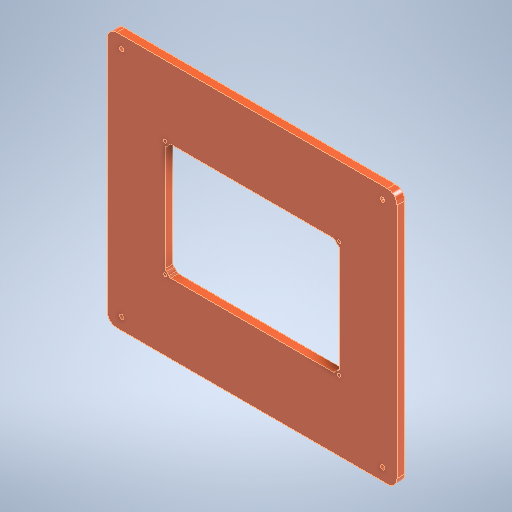
# Autodesk Inventor part: BERÇO GREE
Saved by Autodesk Inventor 2026 (Build 300175050, 175E)
## iProperties
Created: 2025-08-08
Part Number: BERÇO GREE
Material: Genérico
Document SubType Name: Modeling
Designer: Kedson Neves
Density: 1 g/cm^3
Appearance: Suave - Laranja claro
Author: Kedson Neves
Autodesk Inventor part; units mm, degrees
(part 1 of 6)
ref_plane "YZ Plane" through (0, 0, 0) normal (1, 0, 0) x (0, 1, 0)
ref_plane "XZ Plane" through (0, 0, 0) normal (0, 1, 0) x (-1, 0, 0)
ref_plane "XY Plane" through (0, 0, 0) normal (0, 0, 1) x (1, 0, 0)
sketch "Esboço1" plane through (0, 0, 0) normal (0, 0, 1) x (1, 0, 0)
  line L0 (-125.1552, 100.0222) -> (124.8448, 100.0222)
  line L1 (-0.1552, 100.0222) -> (-0.1552, -99.9778)
  line L2 (124.8448, -99.9778) -> (-125.1552, -99.9778)
  line L3 (-150.1552, -132.4778) -> (149.8448, -132.4778)
  line L4 (149.8448, -132.4778) -> (149.8448, 132.5222)
  line L5 (149.8448, 132.5222) -> (-150.1552, 132.5222)
  line L6 (-150.1552, 132.5222) -> (-150.1552, -132.4778)
  line L7 (-150.1552, -132.4778) -> (149.8448, 132.5222) construction
  line L8 (149.8448, -132.4778) -> (-150.1552, 132.5222) construction
  circle A0 centre (-135.1552, 120.0222) radius 1.621
  circle A1 centre (134.8448, 120.0222) radius 1.621
  circle A2 centre (134.8448, -119.9778) radius 1.621
  circle A3 centre (-135.1552, -119.9778) radius 1.621
  point P0 (0, 0)
  point P1 (-0.1552, 0.0222)
  dimension "d0" = 300
  dimension "d1" = 265
  constraints: 18 end point, 4 centre point, 4 midpoint, 2 parallel, 1 horizontal, 1 perpendicular
  measures "d0" distance of L4.end L5.end
  measures "d1" distance of L5.end L3.start
extrude "Extrusão1" add sketch "Esboço1" along normal blind 8
sketch "Esboço2" plane through (0, 0, 8) normal (0, 0, 1) x (1, 0, 0)
  circle A0 centre (-135.1552, 120.0222) radius 1.621 projected
  circle A1 centre (134.8448, 120.0222) radius 1.621 projected
  circle A2 centre (134.8448, -119.9778) radius 1.621 projected
  circle A3 centre (-135.1552, -119.9778) radius 1.621 projected
  point P0 (0, 0)
  constraints: 4 coincident
hole "Furo1" at (-135.1552, 120.0222, 8) at (134.8448, 120.0222, 8) at (134.8448, -119.9778, 8) at (-135.1552, -119.9778, 8) direction (0, 0, -1) diameter 4.5 end through all clearance for "Countersunk Flat Head Screw ISO 2009/7046" size "M4" standard "ISO"
fillet "Arredondamento1" radius 10 4 edges at (-150.1552, -132.4778, 4) (149.8448, -132.4778, 4) (149.8448, 132.5222, 4) (-150.1552, 132.5222, 4)
sketch "Esboço3" plane through (0, 0, 8) normal (0, 0, 1) x (1, 0, 0)
  line L0 (94.8475, -64.9778) -> (94.8475, 65.0222) projected
  line L1 (94.8475, 65.0222) -> (-95.1577, 65.0222) projected
  line L2 (-95.1577, 65.0222) -> (-95.1577, -64.9778) projected
  line L3 (-95.1577, -64.9778) -> (94.8475, -64.9778) projected
  line L4 (91.8485, 60.0222) -> (91.8482, 59.9873) projected
  line L5 (91.8482, 59.9873) -> (91.8473, 59.9524) projected
  line L6 (91.8473, 59.9524) -> (91.8457, 59.9175) projected
  line L7 (91.8457, 59.9175) -> (91.8436, 59.8827) projected
  line L8 (91.8436, 59.8827) -> (91.8409, 59.8479) projected
  line L9 (91.8409, 59.8479) -> (91.8375, 59.8131) projected
  line L10 (91.8375, 59.8131) -> (91.8336, 59.7785) projected
  line L11 (91.8336, 59.7785) -> (91.829, 59.7439) projected
  line L12 (91.829, 59.7439) -> (91.8239, 59.7093) projected
  line L13 (91.8239, 59.7093) -> (91.8181, 59.6749) projected
  line L14 (91.8181, 59.6749) -> (91.8117, 59.6406) projected
  line L15 (91.8117, 59.6406) -> (91.8048, 59.6064) projected
  line L16 (91.8048, 59.6064) -> (91.7972, 59.5723) projected
  line L17 (91.7972, 59.5723) -> (91.7891, 59.5384) projected
  line L18 (91.7891, 59.5384) -> (91.7803, 59.5046) projected
  line L19 (91.7803, 59.5046) -> (91.771, 59.4709) projected
  line L20 (91.771, 59.4709) -> (91.7611, 59.4375) projected
  line L21 (91.7611, 59.4375) -> (91.7506, 59.4042) projected
  line L22 (91.7506, 59.4042) -> (91.7395, 59.3711) projected
  line L23 (91.7395, 59.3711) -> (91.7279, 59.3382) projected
  line L24 (91.7279, 59.3382) -> (91.7156, 59.3055) projected
  line L25 (91.7156, 59.3055) -> (91.7028, 59.273) projected
  line L26 (91.7028, 59.273) -> (91.6895, 59.2407) projected
  line L27 (91.6895, 59.2407) -> (91.6756, 59.2087) projected
  line L28 (91.6756, 59.2087) -> (91.6611, 59.177) projected
  line L29 (91.6611, 59.177) -> (91.6461, 59.1455) projected
  line L30 (91.6461, 59.1455) -> (91.6305, 59.1142) projected
  line L31 (91.6305, 59.1142) -> (91.6144, 59.0833) projected
  line L32 (91.6144, 59.0833) -> (91.5977, 59.0526) projected
  line L33 (91.5977, 59.0526) -> (91.5805, 59.0222) projected
  line L34 (91.5805, 59.0222) -> (91.5628, 58.9921) projected
  line L35 (91.5628, 58.9921) -> (91.5446, 58.9624) projected
  line L36 (91.5446, 58.9624) -> (91.5258, 58.9329) projected
  line L37 (91.5258, 58.9329) -> (91.5066, 58.9038) projected
  line L38 (91.5066, 58.9038) -> (91.4868, 58.8751) projected
  line L39 (91.4868, 58.8751) -> (91.4665, 58.8466) projected
  line L40 (91.4665, 58.8466) -> (91.4458, 58.8186) projected
  line L41 (91.4458, 58.8186) -> (91.4245, 58.7909) projected
  line L42 (91.4245, 58.7909) -> (91.4028, 58.7636) projected
  line L43 (91.4028, 58.7636) -> (91.3806, 58.7366) projected
  line L44 (91.3806, 58.7366) -> (91.3579, 58.7101) projected
  line L45 (91.3579, 58.7101) -> (91.3348, 58.6839) projected
  line L46 (91.3348, 58.6839) -> (91.3112, 58.6582) projected
  line L47 (91.3112, 58.6582) -> (91.2872, 58.6329) projected
  line L48 (91.2872, 58.6329) -> (91.2627, 58.608) projected
  line L49 (91.2627, 58.608) -> (91.2378, 58.5835) projected
  line L50 (91.2378, 58.5835) -> (91.2125, 58.5595) projected
  line L51 (91.2125, 58.5595) -> (91.1867, 58.5359) projected
  line L52 (91.1867, 58.5359) -> (91.1606, 58.5128) projected
  line L53 (91.1606, 58.5128) -> (91.1341, 58.4901) projected
  line L54 (91.1341, 58.4901) -> (91.1071, 58.4679) projected
  line L55 (91.1071, 58.4679) -> (91.0798, 58.4462) projected
  line L56 (91.0798, 58.4462) -> (91.0521, 58.4249) projected
  line L57 (91.0521, 58.4249) -> (91.0241, 58.4042) projected
  line L58 (91.0241, 58.4042) -> (90.9956, 58.3839) projected
  line L59 (90.9956, 58.3839) -> (90.9669, 58.3641) projected
  line L60 (90.9669, 58.3641) -> (90.9378, 58.3449) projected
  line L61 (90.9378, 58.3449) -> (90.9083, 58.3261) projected
  line L62 (90.9083, 58.3261) -> (90.8786, 58.3079) projected
  line L63 (90.8786, 58.3079) -> (90.8485, 58.2902) projected
  line L64 (90.8485, 58.2902) -> (90.8181, 58.273) projected
  line L65 (90.8181, 58.273) -> (90.7874, 58.2563) projected
  line L66 (90.7874, 58.2563) -> (90.7565, 58.2402) projected
  line L67 (90.7565, 58.2402) -> (90.7252, 58.2246) projected
  line L68 (90.7252, 58.2246) -> (90.6937, 58.2096) projected
  line L69 (90.6937, 58.2096) -> (90.662, 58.1951) projected
  line L70 (90.662, 58.1951) -> (90.6299, 58.1812) projected
  line L71 (90.6299, 58.1812) -> (90.5977, 58.1678) projected
  line L72 (90.5977, 58.1678) -> (90.5652, 58.155) projected
  line L73 (90.5652, 58.155) -> (90.5325, 58.1428) projected
  line L74 (90.5325, 58.1428) -> (90.4996, 58.1312) projected
  line L75 (90.4996, 58.1312) -> (90.4665, 58.1201) projected
  line L76 (90.4665, 58.1201) -> (90.4332, 58.1096) projected
  line L77 (90.4332, 58.1096) -> (90.3998, 58.0997) projected
  line L78 (90.3998, 58.0997) -> (90.3661, 58.0904) projected
  line L79 (90.3661, 58.0904) -> (90.3323, 58.0816) projected
  line L80 (90.3323, 58.0816) -> (90.2984, 58.0735) projected
  line L81 (90.2984, 58.0735) -> (90.2643, 58.0659) projected
  line L82 (90.2643, 58.0659) -> (90.2301, 58.059) projected
  line L83 (90.2301, 58.059) -> (90.1958, 58.0526) projected
  line L84 (90.1958, 58.0526) -> (90.1614, 58.0468) projected
  line L85 (90.1614, 58.0468) -> (90.1268, 58.0417) projected
  line L86 (90.1268, 58.0417) -> (90.0922, 58.0371) projected
  line L87 (90.0922, 58.0371) -> (90.0575, 58.0332) projected
  line L88 (90.0575, 58.0332) -> (90.0228, 58.0298) projected
  line L89 (90.0228, 58.0298) -> (89.988, 58.0271) projected
  line L90 (89.988, 58.0271) -> (89.9532, 58.0249) projected
  line L91 (89.9532, 58.0249) -> (89.9183, 58.0234) projected
  line L92 (89.9183, 58.0234) -> (89.8834, 58.0225) projected
  line L93 (89.8834, 58.0225) -> (89.8485, 58.0222) projected
  line L94 (89.8485, 58.0222) -> (89.8136, 58.0225) projected
  line L95 (89.8136, 58.0225) -> (89.7787, 58.0234) projected
  line L96 (89.7787, 58.0234) -> (89.7438, 58.0249) projected
  line L97 (89.7438, 58.0249) -> (89.709, 58.0271) projected
  line L98 (89.709, 58.0271) -> (89.6742, 58.0298) projected
  line L99 (89.6742, 58.0298) -> (89.6394, 58.0332) projected
  line L100 (89.6394, 58.0332) -> (89.6047, 58.0371) projected
  line L101 (89.6047, 58.0371) -> (89.5701, 58.0417) projected
  line L102 (89.5701, 58.0417) -> (89.5356, 58.0468) projected
  line L103 (89.5356, 58.0468) -> (89.5012, 58.0526) projected
  line L104 (89.5012, 58.0526) -> (89.4669, 58.059) projected
  line L105 (89.4669, 58.059) -> (89.4327, 58.0659) projected
  line L106 (89.4327, 58.0659) -> (89.3986, 58.0735) projected
  line L107 (89.3986, 58.0735) -> (89.3646, 58.0816) projected
  line L108 (89.3646, 58.0816) -> (89.3308, 58.0904) projected
  line L109 (89.3308, 58.0904) -> (89.2972, 58.0997) projected
  line L110 (89.2972, 58.0997) -> (89.2637, 58.1096) projected
  line L111 (89.2637, 58.1096) -> (89.2305, 58.1201) projected
  line L112 (89.2305, 58.1201) -> (89.1973, 58.1312) projected
  line L113 (89.1973, 58.1312) -> (89.1644, 58.1428) projected
  line L114 (89.1644, 58.1428) -> (89.1317, 58.155) projected
  line L115 (89.1317, 58.155) -> (89.0993, 58.1678) projected
  line L116 (89.0993, 58.1678) -> (89.067, 58.1812) projected
  line L117 (89.067, 58.1812) -> (89.035, 58.1951) projected
  line L118 (89.035, 58.1951) -> (89.0032, 58.2096) projected
  line L119 (89.0032, 58.2096) -> (88.9717, 58.2246) projected
  line L120 (88.9717, 58.2246) -> (88.9405, 58.2402) projected
  line L121 (88.9405, 58.2402) -> (88.9095, 58.2563) projected
  line L122 (88.9095, 58.2563) -> (88.8789, 58.273) projected
  line L123 (88.8789, 58.273) -> (88.8485, 58.2902) projected
  line L124 (88.8485, 58.2902) -> (88.8184, 58.3079) projected
  line L125 (88.8184, 58.3079) -> (88.7886, 58.3261) projected
  line L126 (88.7886, 58.3261) -> (88.7592, 58.3449) projected
  line L127 (88.7592, 58.3449) -> (88.7301, 58.3641) projected
  line L128 (88.7301, 58.3641) -> (88.7013, 58.3839) projected
  line L129 (88.7013, 58.3839) -> (88.6729, 58.4042) projected
  line L130 (88.6729, 58.4042) -> (88.6449, 58.4249) projected
  line L131 (88.6449, 58.4249) -> (88.6172, 58.4462) projected
  line L132 (88.6172, 58.4462) -> (88.5898, 58.4679) projected
  line L133 (88.5898, 58.4679) -> (88.5629, 58.4901) projected
  line L134 (88.5629, 58.4901) -> (88.5364, 58.5128) projected
  line L135 (88.5364, 58.5128) -> (88.5102, 58.5359) projected
  line L136 (88.5102, 58.5359) -> (88.4845, 58.5595) projected
  line L137 (88.4845, 58.5595) -> (88.4592, 58.5835) projected
  line L138 (88.4592, 58.5835) -> (88.4343, 58.608) projected
  line L139 (88.4343, 58.608) -> (88.4098, 58.6329) projected
  line L140 (88.4098, 58.6329) -> (88.3858, 58.6582) projected
  line L141 (88.3858, 58.6582) -> (88.3622, 58.6839) projected
  line L142 (88.3622, 58.6839) -> (88.3391, 58.7101) projected
  line L143 (88.3391, 58.7101) -> (88.3164, 58.7366) projected
  line L144 (88.3164, 58.7366) -> (88.2942, 58.7636) projected
  line L145 (88.2942, 58.7636) -> (88.2725, 58.7909) projected
  line L146 (88.2725, 58.7909) -> (88.2512, 58.8186) projected
  line L147 (88.2512, 58.8186) -> (88.2305, 58.8466) projected
  line L148 (88.2305, 58.8466) -> (88.2102, 58.8751) projected
  line L149 (88.2102, 58.8751) -> (88.1904, 58.9038) projected
  line L150 (88.1904, 58.9038) -> (88.1711, 58.9329) projected
  line L151 (88.1711, 58.9329) -> (88.1524, 58.9624) projected
  line L152 (88.1524, 58.9624) -> (88.1342, 58.9921) projected
  line L153 (88.1342, 58.9921) -> (88.1164, 59.0222) projected
  line L154 (88.1164, 59.0222) -> (88.0992, 59.0526) projected
  line L155 (88.0992, 59.0526) -> (88.0826, 59.0833) projected
  line L156 (88.0826, 59.0833) -> (88.0665, 59.1142) projected
  line L157 (88.0665, 59.1142) -> (88.0509, 59.1455) projected
  line L158 (88.0509, 59.1455) -> (88.0359, 59.177) projected
  line L159 (88.0359, 59.177) -> (88.0214, 59.2087) projected
  line L160 (88.0214, 59.2087) -> (88.0075, 59.2407) projected
  line L161 (88.0075, 59.2407) -> (87.9941, 59.273) projected
  line L162 (87.9941, 59.273) -> (87.9813, 59.3055) projected
  line L163 (87.9813, 59.3055) -> (87.9691, 59.3382) projected
  line L164 (87.9691, 59.3382) -> (87.9575, 59.3711) projected
  line L165 (87.9575, 59.3711) -> (87.9464, 59.4042) projected
  line L166 (87.9464, 59.4042) -> (87.9359, 59.4375) projected
  line L167 (87.9359, 59.4375) -> (87.926, 59.4709) projected
  line L168 (87.926, 59.4709) -> (87.9166, 59.5046) projected
  line L169 (87.9166, 59.5046) -> (87.9079, 59.5384) projected
  line L170 (87.9079, 59.5384) -> (87.8997, 59.5723) projected
  line L171 (87.8997, 59.5723) -> (87.8922, 59.6064) projected
  line L172 (87.8922, 59.6064) -> (87.8852, 59.6406) projected
  line L173 (87.8852, 59.6406) -> (87.8789, 59.6749) projected
  line L174 (87.8789, 59.6749) -> (87.8731, 59.7093) projected
  line L175 (87.8731, 59.7093) -> (87.868, 59.7439) projected
  line L176 (87.868, 59.7439) -> (87.8634, 59.7785) projected
  line L177 (87.8634, 59.7785) -> (87.8594, 59.8131) projected
  line L178 (87.8594, 59.8131) -> (87.8561, 59.8479) projected
  line L179 (87.8561, 59.8479) -> (87.8534, 59.8827) projected
  line L180 (87.8534, 59.8827) -> (87.8512, 59.9175) projected
  line L181 (87.8512, 59.9175) -> (87.8497, 59.9524) projected
  line L182 (87.8497, 59.9524) -> (87.8488, 59.9873) projected
  line L183 (87.8488, 59.9873) -> (87.8485, 60.0222) projected
  line L184 (87.8485, 60.0222) -> (87.8488, 60.0571) projected
  line L185 (87.8488, 60.0571) -> (87.8497, 60.092) projected
  line L186 (87.8497, 60.092) -> (87.8512, 60.1269) projected
  line L187 (87.8512, 60.1269) -> (87.8534, 60.1617) projected
  line L188 (87.8534, 60.1617) -> (87.8561, 60.1965) projected
  line L189 (87.8561, 60.1965) -> (87.8594, 60.2313) projected
  line L190 (87.8594, 60.2313) -> (87.8634, 60.2659) projected
  line L191 (87.8634, 60.2659) -> (87.868, 60.3005) projected
  line L192 (87.868, 60.3005) -> (87.8731, 60.3351) projected
  line L193 (87.8731, 60.3351) -> (87.8789, 60.3695) projected
  line L194 (87.8789, 60.3695) -> (87.8852, 60.4038) projected
  line L195 (87.8852, 60.4038) -> (87.8922, 60.438) projected
  line L196 (87.8922, 60.438) -> (87.8997, 60.4721) projected
  line L197 (87.8997, 60.4721) -> (87.9079, 60.506) projected
  line L198 (87.9079, 60.506) -> (87.9166, 60.5398) projected
  line L199 (87.9166, 60.5398) -> (87.926, 60.5735) projected
  line L200 (87.926, 60.5735) -> (87.9359, 60.6069) projected
  line L201 (87.9359, 60.6069) -> (87.9464, 60.6402) projected
  line L202 (87.9464, 60.6402) -> (87.9575, 60.6733) projected
  line L203 (87.9575, 60.6733) -> (87.9691, 60.7062) projected
  line L204 (87.9691, 60.7062) -> (87.9813, 60.7389) projected
  line L205 (87.9813, 60.7389) -> (87.9941, 60.7714) projected
  line L206 (87.9941, 60.7714) -> (88.0075, 60.8037) projected
  line L207 (88.0075, 60.8037) -> (88.0214, 60.8357) projected
  line L208 (88.0214, 60.8357) -> (88.0359, 60.8674) projected
  line L209 (88.0359, 60.8674) -> (88.0509, 60.8989) projected
  line L210 (88.0509, 60.8989) -> (88.0665, 60.9302) projected
  line L211 (88.0665, 60.9302) -> (88.0826, 60.9611) projected
  line L212 (88.0826, 60.9611) -> (88.0992, 60.9918) projected
  line L213 (88.0992, 60.9918) -> (88.1164, 61.0222) projected
  line L214 (88.1164, 61.0222) -> (88.1342, 61.0523) projected
  line L215 (88.1342, 61.0523) -> (88.1524, 61.082) projected
  line L216 (88.1524, 61.082) -> (88.1711, 61.1115) projected
  line L217 (88.1711, 61.1115) -> (88.1904, 61.1406) projected
  line L218 (88.1904, 61.1406) -> (88.2102, 61.1694) projected
  line L219 (88.2102, 61.1694) -> (88.2305, 61.1978) projected
  line L220 (88.2305, 61.1978) -> (88.2512, 61.2258) projected
  line L221 (88.2512, 61.2258) -> (88.2725, 61.2535) projected
  line L222 (88.2725, 61.2535) -> (88.2942, 61.2808) projected
  line L223 (88.2942, 61.2808) -> (88.3164, 61.3078) projected
  line L224 (88.3164, 61.3078) -> (88.3391, 61.3343) projected
  line L225 (88.3391, 61.3343) -> (88.3622, 61.3605) projected
  line L226 (88.3622, 61.3605) -> (88.3858, 61.3862) projected
  line L227 (88.3858, 61.3862) -> (88.4098, 61.4115) projected
  line L228 (88.4098, 61.4115) -> (88.4343, 61.4364) projected
  line L229 (88.4343, 61.4364) -> (88.4592, 61.4609) projected
  line L230 (88.4592, 61.4609) -> (88.4845, 61.4849) projected
  line L231 (88.4845, 61.4849) -> (88.5102, 61.5085) projected
  line L232 (88.5102, 61.5085) -> (88.5364, 61.5316) projected
  line L233 (88.5364, 61.5316) -> (88.5629, 61.5543) projected
  line L234 (88.5629, 61.5543) -> (88.5898, 61.5765) projected
  line L235 (88.5898, 61.5765) -> (88.6172, 61.5982) projected
  line L236 (88.6172, 61.5982) -> (88.6449, 61.6195) projected
  line L237 (88.6449, 61.6195) -> (88.6729, 61.6402) projected
  line L238 (88.6729, 61.6402) -> (88.7013, 61.6605) projected
  line L239 (88.7013, 61.6605) -> (88.7301, 61.6803) projected
  line L240 (88.7301, 61.6803) -> (88.7592, 61.6995) projected
  line L241 (88.7592, 61.6995) -> (88.7886, 61.7183) projected
  line L242 (88.7886, 61.7183) -> (88.8184, 61.7365) projected
  line L243 (88.8184, 61.7365) -> (88.8485, 61.7543) projected
  line L244 (88.8485, 61.7543) -> (88.8789, 61.7714) projected
  line L245 (88.8789, 61.7714) -> (88.9095, 61.7881) projected
  line L246 (88.9095, 61.7881) -> (88.9405, 61.8042) projected
  line L247 (88.9405, 61.8042) -> (88.9717, 61.8198) projected
  line L248 (88.9717, 61.8198) -> (89.0032, 61.8348) projected
  line L249 (89.0032, 61.8348) -> (89.035, 61.8493) projected
  line L250 (89.035, 61.8493) -> (89.067, 61.8632) projected
  line L251 (89.067, 61.8632) -> (89.0993, 61.8766) projected
  line L252 (89.0993, 61.8766) -> (89.1317, 61.8894) projected
  line L253 (89.1317, 61.8894) -> (89.1644, 61.9016) projected
  line L254 (89.1644, 61.9016) -> (89.1973, 61.9132) projected
  line L255 (89.1973, 61.9132) -> (89.2305, 61.9243) projected
  line L256 (89.2305, 61.9243) -> (89.2637, 61.9348) projected
  line L257 (89.2637, 61.9348) -> (89.2972, 61.9447) projected
  line L258 (89.2972, 61.9447) -> (89.3308, 61.9541) projected
  line L259 (89.3308, 61.9541) -> (89.3646, 61.9628) projected
  line L260 (89.3646, 61.9628) -> (89.3986, 61.9709) projected
  line L261 (89.3986, 61.9709) -> (89.4327, 61.9785) projected
  line L262 (89.4327, 61.9785) -> (89.4669, 61.9855) projected
  line L263 (89.4669, 61.9855) -> (89.5012, 61.9918) projected
  line L264 (89.5012, 61.9918) -> (89.5356, 61.9976) projected
  line L265 (89.5356, 61.9976) -> (89.5701, 62.0027) projected
  line L266 (89.5701, 62.0027) -> (89.6047, 62.0073) projected
  line L267 (89.6047, 62.0073) -> (89.6394, 62.0112) projected
  line L268 (89.6394, 62.0112) -> (89.6742, 62.0146) projected
  line L269 (89.6742, 62.0146) -> (89.709, 62.0173) projected
  line L270 (89.709, 62.0173) -> (89.7438, 62.0195) projected
  line L271 (89.7438, 62.0195) -> (89.7787, 62.021) projected
  line L272 (89.7787, 62.021) -> (89.8136, 62.0219) projected
  line L273 (89.8136, 62.0219) -> (89.8485, 62.0222) projected
  line L274 (89.8485, 62.0222) -> (89.8834, 62.0219) projected
  line L275 (89.8834, 62.0219) -> (89.9183, 62.021) projected
  line L276 (89.9183, 62.021) -> (89.9532, 62.0195) projected
  line L277 (89.9532, 62.0195) -> (89.988, 62.0173) projected
  line L278 (89.988, 62.0173) -> (90.0228, 62.0146) projected
  line L279 (90.0228, 62.0146) -> (90.0575, 62.0112) projected
  line L280 (90.0575, 62.0112) -> (90.0922, 62.0073) projected
  line L281 (90.0922, 62.0073) -> (90.1268, 62.0027) projected
  line L282 (90.1268, 62.0027) -> (90.1614, 61.9976) projected
  line L283 (90.1614, 61.9976) -> (90.1958, 61.9918) projected
  line L284 (90.1958, 61.9918) -> (90.2301, 61.9855) projected
  line L285 (90.2301, 61.9855) -> (90.2643, 61.9785) projected
  line L286 (90.2643, 61.9785) -> (90.2984, 61.9709) projected
  line L287 (90.2984, 61.9709) -> (90.3323, 61.9628) projected
  line L288 (90.3323, 61.9628) -> (90.3661, 61.9541) projected
  line L289 (90.3661, 61.9541) -> (90.3998, 61.9447) projected
  line L290 (90.3998, 61.9447) -> (90.4332, 61.9348) projected
  line L291 (90.4332, 61.9348) -> (90.4665, 61.9243) projected
  line L292 (90.4665, 61.9243) -> (90.4996, 61.9132) projected
  line L293 (90.4996, 61.9132) -> (90.5325, 61.9016) projected
  line L294 (90.5325, 61.9016) -> (90.5652, 61.8894) projected
  line L295 (90.5652, 61.8894) -> (90.5977, 61.8766) projected
  line L296 (90.5977, 61.8766) -> (90.6299, 61.8632) projected
  line L297 (90.6299, 61.8632) -> (90.662, 61.8493) projected
  line L298 (90.662, 61.8493) -> (90.6937, 61.8348) projected
  line L299 (90.6937, 61.8348) -> (90.7252, 61.8198) projected
  line L300 (90.7252, 61.8198) -> (90.7565, 61.8042) projected
  line L301 (90.7565, 61.8042) -> (90.7874, 61.7881) projected
  line L302 (90.7874, 61.7881) -> (90.8181, 61.7714) projected
  line L303 (90.8181, 61.7714) -> (90.8485, 61.7543) projected
  line L304 (90.8485, 61.7543) -> (90.8786, 61.7365) projected
  line L305 (90.8786, 61.7365) -> (90.9083, 61.7183) projected
  line L306 (90.9083, 61.7183) -> (90.9378, 61.6995) projected
  line L307 (90.9378, 61.6995) -> (90.9669, 61.6803) projected
  line L308 (90.9669, 61.6803) -> (90.9956, 61.6605) projected
  line L309 (90.9956, 61.6605) -> (91.0241, 61.6402) projected
  line L310 (91.0241, 61.6402) -> (91.0521, 61.6195) projected
  line L311 (91.0521, 61.6195) -> (91.0798, 61.5982) projected
  line L312 (91.0798, 61.5982) -> (91.1071, 61.5765) projected
  line L313 (91.1071, 61.5765) -> (91.1341, 61.5543) projected
  line L314 (91.1341, 61.5543) -> (91.1606, 61.5316) projected
  line L315 (91.1606, 61.5316) -> (91.1867, 61.5085) projected
  line L316 (91.1867, 61.5085) -> (91.2125, 61.4849) projected
  line L317 (91.2125, 61.4849) -> (91.2378, 61.4609) projected
  line L318 (91.2378, 61.4609) -> (91.2627, 61.4364) projected
  line L319 (91.2627, 61.4364) -> (91.2872, 61.4115) projected
  line L320 (91.2872, 61.4115) -> (91.3112, 61.3862) projected
  line L321 (91.3112, 61.3862) -> (91.3348, 61.3605) projected
  line L322 (91.3348, 61.3605) -> (91.3579, 61.3343) projected
  line L323 (91.3579, 61.3343) -> (91.3806, 61.3078) projected
  line L324 (91.3806, 61.3078) -> (91.4028, 61.2808) projected
  line L325 (91.4028, 61.2808) -> (91.4245, 61.2535) projected
  line L326 (91.4245, 61.2535) -> (91.4458, 61.2258) projected
  line L327 (91.4458, 61.2258) -> (91.4665, 61.1978) projected
  line L328 (91.4665, 61.1978) -> (91.4868, 61.1694) projected
  line L329 (91.4868, 61.1694) -> (91.5066, 61.1406) projected
  line L330 (91.5066, 61.1406) -> (91.5258, 61.1115) projected
  line L331 (91.5258, 61.1115) -> (91.5446, 61.082) projected
  line L332 (91.5446, 61.082) -> (91.5628, 61.0523) projected
  line L333 (91.5628, 61.0523) -> (91.5805, 61.0222) projected
  line L334 (91.5805, 61.0222) -> (91.5977, 60.9918) projected
  line L335 (91.5977, 60.9918) -> (91.6144, 60.9611) projected
  line L336 (91.6144, 60.9611) -> (91.6305, 60.9302) projected
  line L337 (91.6305, 60.9302) -> (91.6461, 60.8989) projected
  line L338 (91.6461, 60.8989) -> (91.6611, 60.8674) projected
  line L339 (91.6611, 60.8674) -> (91.6756, 60.8357) projected
  line L340 (91.6756, 60.8357) -> (91.6895, 60.8037) projected
  line L341 (91.6895, 60.8037) -> (91.7028, 60.7714) projected
  line L342 (91.7028, 60.7714) -> (91.7156, 60.7389) projected
  line L343 (91.7156, 60.7389) -> (91.7279, 60.7062) projected
  line L344 (91.7279, 60.7062) -> (91.7395, 60.6733) projected
  line L345 (91.7395, 60.6733) -> (91.7506, 60.6402) projected
  line L346 (91.7506, 60.6402) -> (91.7611, 60.6069) projected
  line L347 (91.7611, 60.6069) -> (91.771, 60.5735) projected
  line L348 (91.771, 60.5735) -> (91.7803, 60.5398) projected
  line L349 (91.7803, 60.5398) -> (91.7891, 60.506) projected
  line L350 (91.7891, 60.506) -> (91.7972, 60.4721) projected
  line L351 (91.7972, 60.4721) -> (91.8048, 60.438) projected
  line L352 (91.8048, 60.438) -> (91.8117, 60.4038) projected
  line L353 (91.8117, 60.4038) -> (91.8181, 60.3695) projected
  line L354 (91.8181, 60.3695) -> (91.8239, 60.3351) projected
  line L355 (91.8239, 60.3351) -> (91.829, 60.3005) projected
  line L356 (91.829, 60.3005) -> (91.8336, 60.2659) projected
  line L357 (91.8336, 60.2659) -> (91.8375, 60.2313) projected
  line L358 (91.8375, 60.2313) -> (91.8409, 60.1965) projected
  line L359 (91.8409, 60.1965) -> (91.8436, 60.1617) projected
  line L360 (91.8436, 60.1617) -> (91.8457, 60.1269) projected
  line L361 (91.8457, 60.1269) -> (91.8473, 60.092) projected
  line L362 (91.8473, 60.092) -> (91.8482, 60.0571) projected
  line L363 (91.8482, 60.0571) -> (91.8485, 60.0222) projected
  line L364 (91.8485, -59.9778) -> (91.8482, -60.0127) projected
  line L365 (91.8482, -60.0127) -> (91.8473, -60.0476) projected
  line L366 (91.8473, -60.0476) -> (91.8457, -60.0825) projected
  line L367 (91.8457, -60.0825) -> (91.8436, -60.1173) projected
  line L368 (91.8436, -60.1173) -> (91.8409, -60.1521) projected
  line L369 (91.8409, -60.1521) -> (91.8375, -60.1869) projected
  line L370 (91.8375, -60.1869) -> (91.8336, -60.2215) projected
  line L371 (91.8336, -60.2215) -> (91.829, -60.2562) projected
  line L372 (91.829, -60.2562) -> (91.8239, -60.2907) projected
  line L373 (91.8239, -60.2907) -> (91.8181, -60.3251) projected
  line L374 (91.8181, -60.3251) -> (91.8117, -60.3594) projected
  line L375 (91.8117, -60.3594) -> (91.8048, -60.3936) projected
  line L376 (91.8048, -60.3936) -> (91.7972, -60.4277) projected
  line L377 (91.7972, -60.4277) -> (91.7891, -60.4617) projected
  line L378 (91.7891, -60.4617) -> (91.7803, -60.4954) projected
  line L379 (91.7803, -60.4954) -> (91.771, -60.5291) projected
  line L380 (91.771, -60.5291) -> (91.7611, -60.5626) projected
  line L381 (91.7611, -60.5626) -> (91.7506, -60.5958) projected
  line L382 (91.7506, -60.5958) -> (91.7395, -60.6289) projected
  line L383 (91.7395, -60.6289) -> (91.7279, -60.6618) projected
  line L384 (91.7279, -60.6618) -> (91.7156, -60.6945) projected
  line L385 (91.7156, -60.6945) -> (91.7028, -60.727) projected
  line L386 (91.7028, -60.727) -> (91.6895, -60.7593) projected
  line L387 (91.6895, -60.7593) -> (91.6756, -60.7913) projected
  line L388 (91.6756, -60.7913) -> (91.6611, -60.823) projected
  line L389 (91.6611, -60.823) -> (91.6461, -60.8546) projected
  line L390 (91.6461, -60.8546) -> (91.6305, -60.8858) projected
  line L391 (91.6305, -60.8858) -> (91.6144, -60.9168) projected
  line L392 (91.6144, -60.9168) -> (91.5977, -60.9474) projected
  line L393 (91.5977, -60.9474) -> (91.5805, -60.9778) projected
  line L394 (91.5805, -60.9778) -> (91.5628, -61.0079) projected
  line L395 (91.5628, -61.0079) -> (91.5446, -61.0376) projected
  line L396 (91.5446, -61.0376) -> (91.5258, -61.0671) projected
  line L397 (91.5258, -61.0671) -> (91.5066, -61.0962) projected
  line L398 (91.5066, -61.0962) -> (91.4868, -61.125) projected
  line L399 (91.4868, -61.125) -> (91.4665, -61.1534) projected
  line L400 (91.4665, -61.1534) -> (91.4458, -61.1814) projected
  line L401 (91.4458, -61.1814) -> (91.4245, -61.2091) projected
  line L402 (91.4245, -61.2091) -> (91.4028, -61.2364) projected
  line L403 (91.4028, -61.2364) -> (91.3806, -61.2634) projected
  line L404 (91.3806, -61.2634) -> (91.3579, -61.2899) projected
  line L405 (91.3579, -61.2899) -> (91.3348, -61.3161) projected
  line L406 (91.3348, -61.3161) -> (91.3112, -61.3418) projected
  line L407 (91.3112, -61.3418) -> (91.2872, -61.3671) projected
  line L408 (91.2872, -61.3671) -> (91.2627, -61.392) projected
  line L409 (91.2627, -61.392) -> (91.2378, -61.4165) projected
  line L410 (91.2378, -61.4165) -> (91.2125, -61.4405) projected
  line L411 (91.2125, -61.4405) -> (91.1867, -61.4641) projected
  line L412 (91.1867, -61.4641) -> (91.1606, -61.4872) projected
  line L413 (91.1606, -61.4872) -> (91.1341, -61.5099) projected
  line L414 (91.1341, -61.5099) -> (91.1071, -61.5321) projected
  line L415 (91.1071, -61.5321) -> (91.0798, -61.5538) projected
  line L416 (91.0798, -61.5538) -> (91.0521, -61.5751) projected
  line L417 (91.0521, -61.5751) -> (91.0241, -61.5958) projected
  line L418 (91.0241, -61.5958) -> (90.9956, -61.6161) projected
  line L419 (90.9956, -61.6161) -> (90.9669, -61.6359) projected
  line L420 (90.9669, -61.6359) -> (90.9378, -61.6551) projected
  line L421 (90.9378, -61.6551) -> (90.9083, -61.6739) projected
  line L422 (90.9083, -61.6739) -> (90.8786, -61.6921) projected
  line L423 (90.8786, -61.6921) -> (90.8485, -61.7099) projected
  line L424 (90.8485, -61.7099) -> (90.8181, -61.727) projected
  line L425 (90.8181, -61.727) -> (90.7874, -61.7437) projected
  line L426 (90.7874, -61.7437) -> (90.7565, -61.7598) projected
  line L427 (90.7565, -61.7598) -> (90.7252, -61.7754) projected
  line L428 (90.7252, -61.7754) -> (90.6937, -61.7904) projected
  line L429 (90.6937, -61.7904) -> (90.662, -61.8049) projected
  line L430 (90.662, -61.8049) -> (90.6299, -61.8188) projected
  line L431 (90.6299, -61.8188) -> (90.5977, -61.8322) projected
  line L432 (90.5977, -61.8322) -> (90.5652, -61.845) projected
  line L433 (90.5652, -61.845) -> (90.5325, -61.8572) projected
  line L434 (90.5325, -61.8572) -> (90.4996, -61.8688) projected
  line L435 (90.4996, -61.8688) -> (90.4665, -61.8799) projected
  line L436 (90.4665, -61.8799) -> (90.4332, -61.8904) projected
  line L437 (90.4332, -61.8904) -> (90.3998, -61.9003) projected
  line L438 (90.3998, -61.9003) -> (90.3661, -61.9097) projected
  line L439 (90.3661, -61.9097) -> (90.3323, -61.9184) projected
  line L440 (90.3323, -61.9184) -> (90.2984, -61.9265) projected
  line L441 (90.2984, -61.9265) -> (90.2643, -61.9341) projected
  line L442 (90.2643, -61.9341) -> (90.2301, -61.9411) projected
  line L443 (90.2301, -61.9411) -> (90.1958, -61.9474) projected
  line L444 (90.1958, -61.9474) -> (90.1614, -61.9532) projected
  line L445 (90.1614, -61.9532) -> (90.1268, -61.9583) projected
  line L446 (90.1268, -61.9583) -> (90.0922, -61.9629) projected
  line L447 (90.0922, -61.9629) -> (90.0575, -61.9668) projected
  line L448 (90.0575, -61.9668) -> (90.0228, -61.9702) projected
  line L449 (90.0228, -61.9702) -> (89.988, -61.9729) projected
  line L450 (89.988, -61.9729) -> (89.9532, -61.9751) projected
  line L451 (89.9532, -61.9751) -> (89.9183, -61.9766) projected
  line L452 (89.9183, -61.9766) -> (89.8834, -61.9775) projected
  line L453 (89.8834, -61.9775) -> (89.8485, -61.9778) projected
  line L454 (89.8485, -61.9778) -> (89.8136, -61.9775) projected
  line L455 (89.8136, -61.9775) -> (89.7787, -61.9766) projected
  line L456 (89.7787, -61.9766) -> (89.7438, -61.9751) projected
  line L457 (89.7438, -61.9751) -> (89.709, -61.9729) projected
  line L458 (89.709, -61.9729) -> (89.6742, -61.9702) projected
  line L459 (89.6742, -61.9702) -> (89.6394, -61.9668) projected
  line L460 (89.6394, -61.9668) -> (89.6047, -61.9629) projected
  line L461 (89.6047, -61.9629) -> (89.5701, -61.9583) projected
  line L462 (89.5701, -61.9583) -> (89.5356, -61.9532) projected
  line L463 (89.5356, -61.9532) -> (89.5012, -61.9474) projected
  line L464 (89.5012, -61.9474) -> (89.4669, -61.9411) projected
  line L465 (89.4669, -61.9411) -> (89.4327, -61.9341) projected
  line L466 (89.4327, -61.9341) -> (89.3986, -61.9265) projected
  line L467 (89.3986, -61.9265) -> (89.3646, -61.9184) projected
  line L468 (89.3646, -61.9184) -> (89.3308, -61.9097) projected
  line L469 (89.3308, -61.9097) -> (89.2972, -61.9003) projected
  line L470 (89.2972, -61.9003) -> (89.2637, -61.8904) projected
  line L471 (89.2637, -61.8904) -> (89.2305, -61.8799) projected
  line L472 (89.2305, -61.8799) -> (89.1973, -61.8688) projected
  line L473 (89.1973, -61.8688) -> (89.1644, -61.8572) projected
  line L474 (89.1644, -61.8572) -> (89.1317, -61.845) projected
  line L475 (89.1317, -61.845) -> (89.0993, -61.8322) projected
  line L476 (89.0993, -61.8322) -> (89.067, -61.8188) projected
  line L477 (89.067, -61.8188) -> (89.035, -61.8049) projected
  line L478 (89.035, -61.8049) -> (89.0032, -61.7904) projected
  line L479 (89.0032, -61.7904) -> (88.9717, -61.7754) projected
  line L480 (88.9717, -61.7754) -> (88.9405, -61.7598) projected
  line L481 (88.9405, -61.7598) -> (88.9095, -61.7437) projected
  line L482 (88.9095, -61.7437) -> (88.8789, -61.727) projected
  line L483 (88.8789, -61.727) -> (88.8485, -61.7099) projected
  line L484 (88.8485, -61.7099) -> (88.8184, -61.6921) projected
  line L485 (88.8184, -61.6921) -> (88.7886, -61.6739) projected
  line L486 (88.7886, -61.6739) -> (88.7592, -61.6551) projected
  line L487 (88.7592, -61.6551) -> (88.7301, -61.6359) projected
  line L488 (88.7301, -61.6359) -> (88.7013, -61.6161) projected
  line L489 (88.7013, -61.6161) -> (88.6729, -61.5958) projected
  line L490 (88.6729, -61.5958) -> (88.6449, -61.5751) projected
  line L491 (88.6449, -61.5751) -> (88.6172, -61.5538) projected
  line L492 (88.6172, -61.5538) -> (88.5898, -61.5321) projected
  line L493 (88.5898, -61.5321) -> (88.5629, -61.5099) projected
  line L494 (88.5629, -61.5099) -> (88.5364, -61.4872) projected
  line L495 (88.5364, -61.4872) -> (88.5102, -61.4641) projected
  line L496 (88.5102, -61.4641) -> (88.4845, -61.4405) projected
  line L497 (88.4845, -61.4405) -> (88.4592, -61.4165) projected
  line L498 (88.4592, -61.4165) -> (88.4343, -61.392) projected
  line L499 (88.4343, -61.392) -> (88.4098, -61.3671) projected
  line L500 (88.4098, -61.3671) -> (88.3858, -61.3418) projected
  line L501 (88.3858, -61.3418) -> (88.3622, -61.3161) projected
  line L502 (88.3622, -61.3161) -> (88.3391, -61.2899) projected
  line L503 (88.3391, -61.2899) -> (88.3164, -61.2634) projected
  line L504 (88.3164, -61.2634) -> (88.2942, -61.2364) projected
  line L505 (88.2942, -61.2364) -> (88.2725, -61.2091) projected
  line L506 (88.2725, -61.2091) -> (88.2512, -61.1814) projected
  line L507 (88.2512, -61.1814) -> (88.2305, -61.1534) projected
  line L508 (88.2305, -61.1534) -> (88.2102, -61.125) projected
  line L509 (88.2102, -61.125) -> (88.1904, -61.0962) projected
  line L510 (88.1904, -61.0962) -> (88.1711, -61.0671) projected
  line L511 (88.1711, -61.0671) -> (88.1524, -61.0376) projected
  line L512 (88.1524, -61.0376) -> (88.1342, -61.0079) projected
  line L513 (88.1342, -61.0079) -> (88.1164, -60.9778) projected
  line L514 (88.1164, -60.9778) -> (88.0992, -60.9474) projected
  line L515 (88.0992, -60.9474) -> (88.0826, -60.9168) projected
  line L516 (88.0826, -60.9168) -> (88.0665, -60.8858) projected
  line L517 (88.0665, -60.8858) -> (88.0509, -60.8546) projected
  line L518 (88.0509, -60.8546) -> (88.0359, -60.823) projected
  line L519 (88.0359, -60.823) -> (88.0214, -60.7913) projected
  line L520 (88.0214, -60.7913) -> (88.0075, -60.7593) projected
  line L521 (88.0075, -60.7593) -> (87.9941, -60.727) projected
  line L522 (87.9941, -60.727) -> (87.9813, -60.6945) projected
  line L523 (87.9813, -60.6945) -> (87.9691, -60.6618) projected
  line L524 (87.9691, -60.6618) -> (87.9575, -60.6289) projected
  line L525 (87.9575, -60.6289) -> (87.9464, -60.5958) projected
  line L526 (87.9464, -60.5958) -> (87.9359, -60.5626) projected
  line L527 (87.9359, -60.5626) -> (87.926, -60.5291) projected
  line L528 (87.926, -60.5291) -> (87.9166, -60.4954) projected
  line L529 (87.9166, -60.4954) -> (87.9079, -60.4617) projected
  line L530 (87.9079, -60.4617) -> (87.8997, -60.4277) projected
  line L531 (87.8997, -60.4277) -> (87.8922, -60.3936) projected
  line L532 (87.8922, -60.3936) -> (87.8852, -60.3594) projected
  line L533 (87.8852, -60.3594) -> (87.8789, -60.3251) projected
  line L534 (87.8789, -60.3251) -> (87.8731, -60.2907) projected
  line L535 (87.8731, -60.2907) -> (87.868, -60.2562) projected
  line L536 (87.868, -60.2562) -> (87.8634, -60.2215) projected
  line L537 (87.8634, -60.2215) -> (87.8594, -60.1869) projected
  line L538 (87.8594, -60.1869) -> (87.8561, -60.1521) projected
  line L539 (87.8561, -60.1521) -> (87.8534, -60.1173) projected
  line L540 (87.8534, -60.1173) -> (87.8512, -60.0825) projected
  line L541 (87.8512, -60.0825) -> (87.8497, -60.0476) projected
  line L542 (87.8497, -60.0476) -> (87.8488, -60.0127) projected
  line L543 (87.8488, -60.0127) -> (87.8485, -59.9778) projected
  line L544 (87.8485, -59.9778) -> (87.8488, -59.9429) projected
  line L545 (87.8488, -59.9429) -> (87.8497, -59.908) projected
  line L546 (87.8497, -59.908) -> (87.8512, -59.8731) projected
  line L547 (87.8512, -59.8731) -> (87.8534, -59.8383) projected
  line L548 (87.8534, -59.8383) -> (87.8561, -59.8035) projected
  line L549 (87.8561, -59.8035) -> (87.8594, -59.7688) projected
  line L550 (87.8594, -59.7688) -> (87.8634, -59.7341) projected
  line L551 (87.8634, -59.7341) -> (87.868, -59.6995) projected
  line L552 (87.868, -59.6995) -> (87.8731, -59.6649) projected
  line L553 (87.8731, -59.6649) -> (87.8789, -59.6305) projected
  line L554 (87.8789, -59.6305) -> (87.8852, -59.5962) projected
  line L555 (87.8852, -59.5962) -> (87.8922, -59.562) projected
  line L556 (87.8922, -59.562) -> (87.8997, -59.5279) projected
  line L557 (87.8997, -59.5279) -> (87.9079, -59.494) projected
  line L558 (87.9079, -59.494) -> (87.9166, -59.4602) projected
  line L559 (87.9166, -59.4602) -> (87.926, -59.4265) projected
  line L560 (87.926, -59.4265) -> (87.9359, -59.3931) projected
  line L561 (87.9359, -59.3931) -> (87.9464, -59.3598) projected
  line L562 (87.9464, -59.3598) -> (87.9575, -59.3267) projected
  line L563 (87.9575, -59.3267) -> (87.9691, -59.2938) projected
  line L564 (87.9691, -59.2938) -> (87.9813, -59.2611) projected
  line L565 (87.9813, -59.2611) -> (87.9941, -59.2286) projected
  line L566 (87.9941, -59.2286) -> (88.0075, -59.1963) projected
  line L567 (88.0075, -59.1963) -> (88.0214, -59.1643) projected
  line L568 (88.0214, -59.1643) -> (88.0359, -59.1326) projected
  line L569 (88.0359, -59.1326) -> (88.0509, -59.1011) projected
  line L570 (88.0509, -59.1011) -> (88.0665, -59.0698) projected
  line L571 (88.0665, -59.0698) -> (88.0826, -59.0389) projected
  line L572 (88.0826, -59.0389) -> (88.0992, -59.0082) projected
  line L573 (88.0992, -59.0082) -> (88.1164, -58.9778) projected
  line L574 (88.1164, -58.9778) -> (88.1342, -58.9477) projected
  line L575 (88.1342, -58.9477) -> (88.1524, -58.918) projected
  line L576 (88.1524, -58.918) -> (88.1711, -58.8885) projected
  line L577 (88.1711, -58.8885) -> (88.1904, -58.8594) projected
  line L578 (88.1904, -58.8594) -> (88.2102, -58.8307) projected
  line L579 (88.2102, -58.8307) -> (88.2305, -58.8022) projected
  line L580 (88.2305, -58.8022) -> (88.2512, -58.7742) projected
  line L581 (88.2512, -58.7742) -> (88.2725, -58.7465) projected
  line L582 (88.2725, -58.7465) -> (88.2942, -58.7192) projected
  line L583 (88.2942, -58.7192) -> (88.3164, -58.6922) projected
  line L584 (88.3164, -58.6922) -> (88.3391, -58.6657) projected
  line L585 (88.3391, -58.6657) -> (88.3622, -58.6396) projected
  line L586 (88.3622, -58.6396) -> (88.3858, -58.6138) projected
  line L587 (88.3858, -58.6138) -> (88.4098, -58.5885) projected
  line L588 (88.4098, -58.5885) -> (88.4343, -58.5636) projected
  line L589 (88.4343, -58.5636) -> (88.4592, -58.5391) projected
  line L590 (88.4592, -58.5391) -> (88.4845, -58.5151) projected
  line L591 (88.4845, -58.5151) -> (88.5102, -58.4915) projected
  line L592 (88.5102, -58.4915) -> (88.5364, -58.4684) projected
  line L593 (88.5364, -58.4684) -> (88.5629, -58.4457) projected
  line L594 (88.5629, -58.4457) -> (88.5898, -58.4235) projected
  line L595 (88.5898, -58.4235) -> (88.6172, -58.4018) projected
  line L596 (88.6172, -58.4018) -> (88.6449, -58.3805) projected
  line L597 (88.6449, -58.3805) -> (88.6729, -58.3598) projected
  line L598 (88.6729, -58.3598) -> (88.7013, -58.3395) projected
  line L599 (88.7013, -58.3395) -> (88.7301, -58.3197) projected
  line L600 (88.7301, -58.3197) -> (88.7592, -58.3005) projected
  line L601 (88.7592, -58.3005) -> (88.7886, -58.2817) projected
  line L602 (88.7886, -58.2817) -> (88.8184, -58.2635) projected
  line L603 (88.8184, -58.2635) -> (88.8485, -58.2458) projected
  line L604 (88.8485, -58.2458) -> (88.8789, -58.2286) projected
  line L605 (88.8789, -58.2286) -> (88.9095, -58.2119) projected
  line L606 (88.9095, -58.2119) -> (88.9405, -58.1958) projected
  line L607 (88.9405, -58.1958) -> (88.9717, -58.1802) projected
  line L608 (88.9717, -58.1802) -> (89.0032, -58.1652) projected
  line L609 (89.0032, -58.1652) -> (89.035, -58.1507) projected
  line L610 (89.035, -58.1507) -> (89.067, -58.1368) projected
  line L611 (89.067, -58.1368) -> (89.0993, -58.1234) projected
  line L612 (89.0993, -58.1234) -> (89.1317, -58.1107) projected
  line L613 (89.1317, -58.1107) -> (89.1644, -58.0984) projected
  line L614 (89.1644, -58.0984) -> (89.1973, -58.0868) projected
  line L615 (89.1973, -58.0868) -> (89.2305, -58.0757) projected
  line L616 (89.2305, -58.0757) -> (89.2637, -58.0652) projected
  line L617 (89.2637, -58.0652) -> (89.2972, -58.0553) projected
  line L618 (89.2972, -58.0553) -> (89.3308, -58.046) projected
  line L619 (89.3308, -58.046) -> (89.3646, -58.0372) projected
  line L620 (89.3646, -58.0372) -> (89.3986, -58.0291) projected
  line L621 (89.3986, -58.0291) -> (89.4327, -58.0215) projected
  line L622 (89.4327, -58.0215) -> (89.4669, -58.0146) projected
  line L623 (89.4669, -58.0146) -> (89.5012, -58.0082) projected
  line L624 (89.5012, -58.0082) -> (89.5356, -58.0024) projected
  line L625 (89.5356, -58.0024) -> (89.5701, -57.9973) projected
  line L626 (89.5701, -57.9973) -> (89.6047, -57.9927) projected
  line L627 (89.6047, -57.9927) -> (89.6394, -57.9888) projected
  line L628 (89.6394, -57.9888) -> (89.6742, -57.9854) projected
  line L629 (89.6742, -57.9854) -> (89.709, -57.9827) projected
  line L630 (89.709, -57.9827) -> (89.7438, -57.9806) projected
  line L631 (89.7438, -57.9806) -> (89.7787, -57.979) projected
  line L632 (89.7787, -57.979) -> (89.8136, -57.9781) projected
  line L633 (89.8136, -57.9781) -> (89.8485, -57.9778) projected
  line L634 (89.8485, -57.9778) -> (89.8834, -57.9781) projected
  line L635 (89.8834, -57.9781) -> (89.9183, -57.979) projected
  line L636 (89.9183, -57.979) -> (89.9532, -57.9806) projected
  line L637 (89.9532, -57.9806) -> (89.988, -57.9827) projected
  line L638 (89.988, -57.9827) -> (90.0228, -57.9854) projected
  line L639 (90.0228, -57.9854) -> (90.0575, -57.9888) projected
  line L640 (90.0575, -57.9888) -> (90.0922, -57.9927) projected
  line L641 (90.0922, -57.9927) -> (90.1268, -57.9973) projected
  line L642 (90.1268, -57.9973) -> (90.1614, -58.0024) projected
  line L643 (90.1614, -58.0024) -> (90.1958, -58.0082) projected
  line L644 (90.1958, -58.0082) -> (90.2301, -58.0146) projected
  line L645 (90.2301, -58.0146) -> (90.2643, -58.0215) projected
  line L646 (90.2643, -58.0215) -> (90.2984, -58.0291) projected
  line L647 (90.2984, -58.0291) -> (90.3323, -58.0372) projected
  line L648 (90.3323, -58.0372) -> (90.3661, -58.046) projected
  line L649 (90.3661, -58.046) -> (90.3998, -58.0553) projected
  line L650 (90.3998, -58.0553) -> (90.4332, -58.0652) projected
  line L651 (90.4332, -58.0652) -> (90.4665, -58.0757) projected
  line L652 (90.4665, -58.0757) -> (90.4996, -58.0868) projected
  line L653 (90.4996, -58.0868) -> (90.5325, -58.0984) projected
  line L654 (90.5325, -58.0984) -> (90.5652, -58.1107) projected
  line L655 (90.5652, -58.1107) -> (90.5977, -58.1234) projected
  line L656 (90.5977, -58.1234) -> (90.6299, -58.1368) projected
  line L657 (90.6299, -58.1368) -> (90.662, -58.1507) projected
  line L658 (90.662, -58.1507) -> (90.6937, -58.1652) projected
  line L659 (90.6937, -58.1652) -> (90.7252, -58.1802) projected
  line L660 (90.7252, -58.1802) -> (90.7565, -58.1958) projected
  line L661 (90.7565, -58.1958) -> (90.7874, -58.2119) projected
  line L662 (90.7874, -58.2119) -> (90.8181, -58.2286) projected
  line L663 (90.8181, -58.2286) -> (90.8485, -58.2458) projected
  line L664 (90.8485, -58.2458) -> (90.8786, -58.2635) projected
  line L665 (90.8786, -58.2635) -> (90.9083, -58.2817) projected
  line L666 (90.9083, -58.2817) -> (90.9378, -58.3005) projected
  line L667 (90.9378, -58.3005) -> (90.9669, -58.3197) projected
  line L668 (90.9669, -58.3197) -> (90.9956, -58.3395) projected
  line L669 (90.9956, -58.3395) -> (91.0241, -58.3598) projected
  line L670 (91.0241, -58.3598) -> (91.0521, -58.3805) projected
  line L671 (91.0521, -58.3805) -> (91.0798, -58.4018) projected
  line L672 (91.0798, -58.4018) -> (91.1071, -58.4235) projected
  line L673 (91.1071, -58.4235) -> (91.1341, -58.4457) projected
  line L674 (91.1341, -58.4457) -> (91.1606, -58.4684) projected
  line L675 (91.1606, -58.4684) -> (91.1867, -58.4915) projected
  line L676 (91.1867, -58.4915) -> (91.2125, -58.5151) projected
  line L677 (91.2125, -58.5151) -> (91.2378, -58.5391) projected
  line L678 (91.2378, -58.5391) -> (91.2627, -58.5636) projected
  line L679 (91.2627, -58.5636) -> (91.2872, -58.5885) projected
  line L680 (91.2872, -58.5885) -> (91.3112, -58.6138) projected
  line L681 (91.3112, -58.6138) -> (91.3348, -58.6396) projected
  line L682 (91.3348, -58.6396) -> (91.3579, -58.6657) projected
  line L683 (91.3579, -58.6657) -> (91.3806, -58.6922) projected
  line L684 (91.3806, -58.6922) -> (91.4028, -58.7192) projected
  line L685 (91.4028, -58.7192) -> (91.4245, -58.7465) projected
  line L686 (91.4245, -58.7465) -> (91.4458, -58.7742) projected
  line L687 (91.4458, -58.7742) -> (91.4665, -58.8022) projected
  line L688 (91.4665, -58.8022) -> (91.4868, -58.8307) projected
  line L689 (91.4868, -58.8307) -> (91.5066, -58.8594) projected
  line L690 (91.5066, -58.8594) -> (91.5258, -58.8885) projected
  line L691 (91.5258, -58.8885) -> (91.5446, -58.918) projected
  line L692 (91.5446, -58.918) -> (91.5628, -58.9477) projected
  line L693 (91.5628, -58.9477) -> (91.5805, -58.9778) projected
  line L694 (91.5805, -58.9778) -> (91.5977, -59.0082) projected
  line L695 (91.5977, -59.0082) -> (91.6144, -59.0389) projected
  line L696 (91.6144, -59.0389) -> (91.6305, -59.0698) projected
  line L697 (91.6305, -59.0698) -> (91.6461, -59.1011) projected
  line L698 (91.6461, -59.1011) -> (91.6611, -59.1326) projected
  line L699 (91.6611, -59.1326) -> (91.6756, -59.1643) projected
  line L700 (91.6756, -59.1643) -> (91.6895, -59.1963) projected
  line L701 (91.6895, -59.1963) -> (91.7028, -59.2286) projected
  line L702 (91.7028, -59.2286) -> (91.7156, -59.2611) projected
  line L703 (91.7156, -59.2611) -> (91.7279, -59.2938) projected
  line L704 (91.7279, -59.2938) -> (91.7395, -59.3267) projected
  line L705 (91.7395, -59.3267) -> (91.7506, -59.3598) projected
  line L706 (91.7506, -59.3598) -> (91.7611, -59.3931) projected
  line L707 (91.7611, -59.3931) -> (91.771, -59.4265) projected
  line L708 (91.771, -59.4265) -> (91.7803, -59.4602) projected
  line L709 (91.7803, -59.4602) -> (91.7891, -59.494) projected
  line L710 (91.7891, -59.494) -> (91.7972, -59.5279) projected
  line L711 (91.7972, -59.5279) -> (91.8048, -59.562) projected
  line L712 (91.8048, -59.562) -> (91.8117, -59.5962) projected
  line L713 (91.8117, -59.5962) -> (91.8181, -59.6305) projected
  line L714 (91.8181, -59.6305) -> (91.8239, -59.6649) projected
  line L715 (91.8239, -59.6649) -> (91.829, -59.6995) projected
  line L716 (91.829, -59.6995) -> (91.8336, -59.7341) projected
  line L717 (91.8336, -59.7341) -> (91.8375, -59.7688) projected
  line L718 (91.8375, -59.7688) -> (91.8409, -59.8035) projected
  line L719 (91.8409, -59.8035) -> (91.8436, -59.8383) projected
  line L720 (91.8436, -59.8383) -> (91.8457, -59.8731) projected
  line L721 (91.8457, -59.8731) -> (91.8473, -59.908) projected
  line L722 (91.8473, -59.908) -> (91.8482, -59.9429) projected
  line L723 (91.8482, -59.9429) -> (91.8485, -59.9778) projected
  line L724 (-88.1514, -59.9778) -> (-88.1517, -60.0127) projected
  line L725 (-88.1517, -60.0127) -> (-88.1526, -60.0476) projected
  line L726 (-88.1526, -60.0476) -> (-88.1542, -60.0825) projected
  line L727 (-88.1542, -60.0825) -> (-88.1563, -60.1173) projected
  line L728 (-88.1563, -60.1173) -> (-88.159, -60.1521) projected
  line L729 (-88.159, -60.1521) -> (-88.1624, -60.1869) projected
  line L730 (-88.1624, -60.1869) -> (-88.1663, -60.2215) projected
  line L731 (-88.1663, -60.2215) -> (-88.1709, -60.2562) projected
  line L732 (-88.1709, -60.2562) -> (-88.176, -60.2907) projected
  line L733 (-88.176, -60.2907) -> (-88.1818, -60.3251) projected
  line L734 (-88.1818, -60.3251) -> (-88.1882, -60.3594) projected
  line L735 (-88.1882, -60.3594) -> (-88.1951, -60.3936) projected
  line L736 (-88.1951, -60.3936) -> (-88.2027, -60.4277) projected
  line L737 (-88.2027, -60.4277) -> (-88.2108, -60.4617) projected
  line L738 (-88.2108, -60.4617) -> (-88.2196, -60.4954) projected
  line L739 (-88.2196, -60.4954) -> (-88.2289, -60.5291) projected
  line L740 (-88.2289, -60.5291) -> (-88.2388, -60.5626) projected
  line L741 (-88.2388, -60.5626) -> (-88.2493, -60.5958) projected
  line L742 (-88.2493, -60.5958) -> (-88.2604, -60.6289) projected
  line L743 (-88.2604, -60.6289) -> (-88.272, -60.6618) projected
  line L744 (-88.272, -60.6618) -> (-88.2843, -60.6945) projected
  line L745 (-88.2843, -60.6945) -> (-88.297, -60.727) projected
  line L746 (-88.297, -60.727) -> (-88.3104, -60.7593) projected
  line L747 (-88.3104, -60.7593) -> (-88.3243, -60.7913) projected
  line L748 (-88.3243, -60.7913) -> (-88.3388, -60.823) projected
  line L749 (-88.3388, -60.823) -> (-88.3538, -60.8546) projected
  line L750 (-88.3538, -60.8546) -> (-88.3694, -60.8858) projected
  line L751 (-88.3694, -60.8858) -> (-88.3855, -60.9168) projected
  line L752 (-88.3855, -60.9168) -> (-88.4022, -60.9474) projected
  line L753 (-88.4022, -60.9474) -> (-88.4194, -60.9778) projected
  line L754 (-88.4194, -60.9778) -> (-88.4371, -61.0079) projected
  line L755 (-88.4371, -61.0079) -> (-88.4553, -61.0376) projected
  line L756 (-88.4553, -61.0376) -> (-88.4741, -61.0671) projected
  line L757 (-88.4741, -61.0671) -> (-88.4933, -61.0962) projected
  line L758 (-88.4933, -61.0962) -> (-88.5131, -61.125) projected
  line L759 (-88.5131, -61.125) -> (-88.5334, -61.1534) projected
  line L760 (-88.5334, -61.1534) -> (-88.5541, -61.1814) projected
  line L761 (-88.5541, -61.1814) -> (-88.5754, -61.2091) projected
  line L762 (-88.5754, -61.2091) -> (-88.5971, -61.2364) projected
  line L763 (-88.5971, -61.2364) -> (-88.6193, -61.2634) projected
  line L764 (-88.6193, -61.2634) -> (-88.642, -61.2899) projected
  line L765 (-88.642, -61.2899) -> (-88.6651, -61.3161) projected
  line L766 (-88.6651, -61.3161) -> (-88.6887, -61.3418) projected
  line L767 (-88.6887, -61.3418) -> (-88.7127, -61.3671) projected
  line L768 (-88.7127, -61.3671) -> (-88.7372, -61.392) projected
  line L769 (-88.7372, -61.392) -> (-88.7621, -61.4165) projected
  line L770 (-88.7621, -61.4165) -> (-88.7874, -61.4405) projected
  line L771 (-88.7874, -61.4405) -> (-88.8132, -61.4641) projected
  line L772 (-88.8132, -61.4641) -> (-88.8393, -61.4872) projected
  line L773 (-88.8393, -61.4872) -> (-88.8658, -61.5099) projected
  line L774 (-88.8658, -61.5099) -> (-88.8928, -61.5321) projected
  line L775 (-88.8928, -61.5321) -> (-88.9201, -61.5538) projected
  line L776 (-88.9201, -61.5538) -> (-88.9478, -61.5751) projected
  line L777 (-88.9478, -61.5751) -> (-88.9758, -61.5958) projected
  line L778 (-88.9758, -61.5958) -> (-89.0043, -61.6161) projected
  line L779 (-89.0043, -61.6161) -> (-89.033, -61.6359) projected
  line L780 (-89.033, -61.6359) -> (-89.0621, -61.6551) projected
  line L781 (-89.0621, -61.6551) -> (-89.0916, -61.6739) projected
  line L782 (-89.0916, -61.6739) -> (-89.1213, -61.6921) projected
  line L783 (-89.1213, -61.6921) -> (-89.1514, -61.7099) projected
  line L784 (-89.1514, -61.7099) -> (-89.1818, -61.727) projected
  line L785 (-89.1818, -61.727) -> (-89.2125, -61.7437) projected
  line L786 (-89.2125, -61.7437) -> (-89.2434, -61.7598) projected
  line L787 (-89.2434, -61.7598) -> (-89.2747, -61.7754) projected
  line L788 (-89.2747, -61.7754) -> (-89.3062, -61.7904) projected
  line L789 (-89.3062, -61.7904) -> (-89.3379, -61.8049) projected
  line L790 (-89.3379, -61.8049) -> (-89.3699, -61.8188) projected
  line L791 (-89.3699, -61.8188) -> (-89.4022, -61.8322) projected
  line L792 (-89.4022, -61.8322) -> (-89.4347, -61.845) projected
  line L793 (-89.4347, -61.845) -> (-89.4674, -61.8572) projected
  line L794 (-89.4674, -61.8572) -> (-89.5003, -61.8688) projected
  line L795 (-89.5003, -61.8688) -> (-89.5334, -61.8799) projected
  line L796 (-89.5334, -61.8799) -> (-89.5667, -61.8904) projected
  line L797 (-89.5667, -61.8904) -> (-89.6001, -61.9003) projected
  line L798 (-89.6001, -61.9003) -> (-89.6338, -61.9097) projected
  line L799 (-89.6338, -61.9097) -> (-89.6676, -61.9184) projected
  line L800 (-89.6676, -61.9184) -> (-89.7015, -61.9265) projected
  line L801 (-89.7015, -61.9265) -> (-89.7356, -61.9341) projected
  line L802 (-89.7356, -61.9341) -> (-89.7698, -61.9411) projected
  line L803 (-89.7698, -61.9411) -> (-89.8041, -61.9474) projected
  line L804 (-89.8041, -61.9474) -> (-89.8385, -61.9532) projected
  line L805 (-89.8385, -61.9532) -> (-89.8731, -61.9583) projected
  line L806 (-89.8731, -61.9583) -> (-89.9077, -61.9629) projected
  line L807 (-89.9077, -61.9629) -> (-89.9424, -61.9668) projected
  line L808 (-89.9424, -61.9668) -> (-89.9771, -61.9702) projected
  line L809 (-89.9771, -61.9702) -> (-90.0119, -61.9729) projected
  line L810 (-90.0119, -61.9729) -> (-90.0467, -61.9751) projected
  line L811 (-90.0467, -61.9751) -> (-90.0816, -61.9766) projected
  line L812 (-90.0816, -61.9766) -> (-90.1165, -61.9775) projected
  line L813 (-90.1165, -61.9775) -> (-90.1514, -61.9778) projected
  line L814 (-90.1514, -61.9778) -> (-90.1863, -61.9775) projected
  line L815 (-90.1863, -61.9775) -> (-90.2212, -61.9766) projected
  line L816 (-90.2212, -61.9766) -> (-90.2561, -61.9751) projected
  line L817 (-90.2561, -61.9751) -> (-90.2909, -61.9729) projected
  line L818 (-90.2909, -61.9729) -> (-90.3257, -61.9702) projected
  line L819 (-90.3257, -61.9702) -> (-90.3605, -61.9668) projected
  line L820 (-90.3605, -61.9668) -> (-90.3951, -61.9629) projected
  line L821 (-90.3951, -61.9629) -> (-90.4298, -61.9583) projected
  line L822 (-90.4298, -61.9583) -> (-90.4643, -61.9532) projected
  line L823 (-90.4643, -61.9532) -> (-90.4987, -61.9474) projected
  line L824 (-90.4987, -61.9474) -> (-90.533, -61.9411) projected
  line L825 (-90.533, -61.9411) -> (-90.5672, -61.9341) projected
  line L826 (-90.5672, -61.9341) -> (-90.6013, -61.9265) projected
  line L827 (-90.6013, -61.9265) -> (-90.6353, -61.9184) projected
  line L828 (-90.6353, -61.9184) -> (-90.669, -61.9097) projected
  line L829 (-90.669, -61.9097) -> (-90.7027, -61.9003) projected
  line L830 (-90.7027, -61.9003) -> (-90.7362, -61.8904) projected
  line L831 (-90.7362, -61.8904) -> (-90.7694, -61.8799) projected
  line L832 (-90.7694, -61.8799) -> (-90.8025, -61.8688) projected
  line L833 (-90.8025, -61.8688) -> (-90.8354, -61.8572) projected
  line L834 (-90.8354, -61.8572) -> (-90.8681, -61.845) projected
  line L835 (-90.8681, -61.845) -> (-90.9006, -61.8322) projected
  line L836 (-90.9006, -61.8322) -> (-90.9329, -61.8188) projected
  line L837 (-90.9329, -61.8188) -> (-90.9649, -61.8049) projected
  line L838 (-90.9649, -61.8049) -> (-90.9966, -61.7904) projected
  line L839 (-90.9966, -61.7904) -> (-91.0282, -61.7754) projected
  line L840 (-91.0282, -61.7754) -> (-91.0594, -61.7598) projected
  line L841 (-91.0594, -61.7598) -> (-91.0904, -61.7437) projected
  line L842 (-91.0904, -61.7437) -> (-91.121, -61.727) projected
  line L843 (-91.121, -61.727) -> (-91.1514, -61.7099) projected
  line L844 (-91.1514, -61.7099) -> (-91.1815, -61.6921) projected
  line L845 (-91.1815, -61.6921) -> (-91.2112, -61.6739) projected
  line L846 (-91.2112, -61.6739) -> (-91.2407, -61.6551) projected
  line L847 (-91.2407, -61.6551) -> (-91.2698, -61.6359) projected
  line L848 (-91.2698, -61.6359) -> (-91.2986, -61.6161) projected
  line L849 (-91.2986, -61.6161) -> (-91.327, -61.5958) projected
  line L850 (-91.327, -61.5958) -> (-91.355, -61.5751) projected
  line L851 (-91.355, -61.5751) -> (-91.3827, -61.5538) projected
  line L852 (-91.3827, -61.5538) -> (-91.41, -61.5321) projected
  line L853 (-91.41, -61.5321) -> (-91.437, -61.5099) projected
  line L854 (-91.437, -61.5099) -> (-91.4635, -61.4872) projected
  line L855 (-91.4635, -61.4872) -> (-91.4897, -61.4641) projected
  line L856 (-91.4897, -61.4641) -> (-91.5154, -61.4405) projected
  line L857 (-91.5154, -61.4405) -> (-91.5407, -61.4165) projected
  line L858 (-91.5407, -61.4165) -> (-91.5656, -61.392) projected
  line L859 (-91.5656, -61.392) -> (-91.5901, -61.3671) projected
  line L860 (-91.5901, -61.3671) -> (-91.6141, -61.3418) projected
  line L861 (-91.6141, -61.3418) -> (-91.6377, -61.3161) projected
  line L862 (-91.6377, -61.3161) -> (-91.6608, -61.2899) projected
  line L863 (-91.6608, -61.2899) -> (-91.6835, -61.2634) projected
  line L864 (-91.6835, -61.2634) -> (-91.7057, -61.2364) projected
  line L865 (-91.7057, -61.2364) -> (-91.7274, -61.2091) projected
  line L866 (-91.7274, -61.2091) -> (-91.7487, -61.1814) projected
  line L867 (-91.7487, -61.1814) -> (-91.7694, -61.1534) projected
  line L868 (-91.7694, -61.1534) -> (-91.7897, -61.125) projected
  line L869 (-91.7897, -61.125) -> (-91.8095, -61.0962) projected
  line L870 (-91.8095, -61.0962) -> (-91.8287, -61.0671) projected
  line L871 (-91.8287, -61.0671) -> (-91.8475, -61.0376) projected
  line L872 (-91.8475, -61.0376) -> (-91.8657, -61.0079) projected
  line L873 (-91.8657, -61.0079) -> (-91.8835, -60.9778) projected
  line L874 (-91.8835, -60.9778) -> (-91.9006, -60.9474) projected